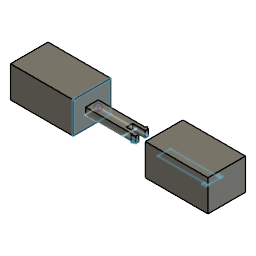
Snap Fit Joint (Autodesk Fusion 360 design; units mm, degrees)
part number: 2026-06-07-14-29-13-328
Autodesk Fusion 360 part; units mm, degrees
sketch "Sketch3" plane through (0, 0, 0) normal (0, 1, 0) x (1, 0, 0)
  line L0 (0, 0) -> (6, 0)
  line L1 (6, 0) -> (6, -2)
  line L2 (6, -2) -> (0, -2)
  line L3 (0, -2) -> (0, 0)
  line L4 (6, 0) -> (8, 0)
  line L5 (8, 0) -> (8, -0.5)
  line L6 (8, -0.5) -> (6, -0.5)
  line L7 (6, -0.5) -> (6, 0)
  line L8 (6, -1.5) -> (8, -1.5)
  line L9 (8, -1.5) -> (8, -2)
  line L10 (8, -2) -> (6, -2)
  line L11 (6, -2) -> (6, -1.5)
  line L12 (7.5, 0) -> (7.5, 0.25)
  line L13 (7.5, 0.25) -> (8, 0)
  line L14 (7.5, -2) -> (7.5, -2.25)
  line L15 (7.5, -2.25) -> (8, -2)
  dimension "d7" = 6
  dimension "d8" = 2
  dimension "d9" = 0.25
  dimension "d10" = 0.25
  constraint horizontal L0
  constraint vertical L1
  constraint horizontal L2
  constraint vertical L3
  constraint coincident L0.start L3.end
  constraint horizontal L4
  constraint vertical L5
  constraint horizontal L6
  constraint vertical L7
  constraint horizontal L8
  constraint vertical L9
  constraint horizontal L10
  constraint vertical L11
  constraint coincident L1 L8.start
  constraint coincident L4 L12.start
  constraint perpendicular L4 L12
  constraint coincident L10 L14.start
  constraint perpendicular L10 L14
  measures "d7" distance of L0.start L0.end
  measures "d8" distance of L0.start L2.end
  measures "d9" distance of L12.start L12.end
  measures "d10" distance of L14.start L14.end
extrude "Extrude3" add sketch "Sketch3" along normal blind 1 makes body 1
sketch "Sketch4" plane through (0, 0, 0) normal (1, 0, 0) x (0, 0, -1)
  line L0 (2, -2) -> (-4, -2)
  line L1 (-4, -2) -> (-4, 3)
  line L2 (-4, 3) -> (2, 3)
  line L3 (2, 3) -> (2, -2)
  constraint horizontal L0
  constraint vertical L1
  constraint horizontal L2
  constraint vertical L3
extrude "Extrude4" add sketch "Sketch4" against normal blind 10 bodies 1
sketch "Sketch5" plane through (0, 0, 0) normal (1, 0, 0) x (0, 0, -1)
  line L0 (-4, 3, 11.5) -> (2, 3, 11.5)
  line L1 (2, 3, 11.5) -> (2, -2, 11.5)
  line L2 (2, -2, 11.5) -> (-4, -2, 11.5)
  line L3 (-4, -2, 11.5) -> (-4, 3, 11.5)
extrude "Extrude5" add sketch "Sketch5" along normal blind 10 separate body contours L0 L1 L2 L3 in plane through (11.5, 0, 0) normal (1, 0, 0) makes body 2
sketch "Sketch7" plane through (0, 0, 0) normal (0, 1, 0) x (1, 0, 0)
  line L0 (19.5, 0) -> (11.5, 0)
  line L1 (11.5, 0) -> (11.5, -2)
  line L2 (11.5, -2) -> (19.5, -2)
  line L3 (19.5, -2) -> (19.5, 0)
  line L4 (19.5, 0) -> (18.9, 0)
  line L5 (18.9, 0) -> (18.9, 0.35)
  line L6 (18.9, 0.35) -> (19.5, 0.35)
  line L7 (19.5, 0.35) -> (19.5, 0)
  line L8 (19.5, -2) -> (18.9, -2)
  line L9 (18.9, -2) -> (18.9, -2.35)
  line L10 (18.9, -2.35) -> (19.5, -2.35)
  line L11 (19.5, -2.35) -> (19.5, -2)
  dimension "d21" = 0.6
  dimension "d22" = 0.35
  dimension "d23" = 0.6
  dimension "d24" = 0.35
  dimension "d27" = 8
  dimension "d28" = 2
  constraint horizontal L0
  constraint vertical L1
  constraint horizontal L2
  constraint vertical L3
  constraint horizontal L4
  constraint vertical L5
  constraint horizontal L6
  constraint vertical L7
  constraint horizontal L8
  constraint vertical L9
  constraint horizontal L10
  constraint vertical L11
  measures "d21" distance of L0.start L4.end
  measures "d22" distance of L0.start L6.end
  measures "d23" distance of L2.end L8.end
  measures "d24" distance of L2.end L10.end
  measures "d27" distance of L1.end L2.end
  measures "d28" distance of L0.end L1.end
extrude "Extrude6" cut sketch "Sketch7" along normal blind 1 bodies 2
extrude "Extrude7" add sketch "Sketch7" along normal blind 1 contours L0 L1 L2 L3 L4 L8 bodies 2
extrude "Extrude8" cut sketch "Sketch7" along normal blind 1 bodies 2
move_face "OffsetFaces1" offset -0.1 7 faces at (16.4333, 0.3333, 0) (19.5, 0.3333, 1.45) (13.9667, 0.3333, 2) (13.9667, 1, 0.6667) (19.1, 0.3333, 2.35) (13.9667, 0, 0.6667) (19.1, 0.3333, -0.35) on bodies 2
